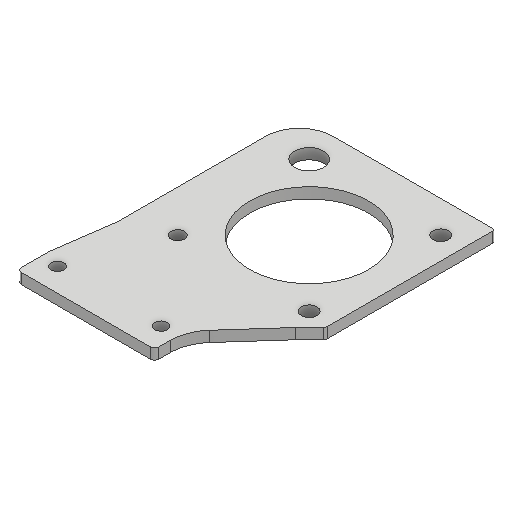
# Autodesk Inventor part: 3DP_ABS_E3D_Titan_Mounting_Plate
Saved by Autodesk Inventor 2026.1 (Build 301233000, 233)
## iProperties
Created: 2017-07-28
Part Number: 3DP_ABS_E3D_Titan_Mounting_Plate
Material: Ogólny
Document SubType Name: Modeling
Designer: Andrzej
Density: 1 g/cm^3
Appearance: Domyślna
Author: Andrzej
Autodesk Inventor part; units mm, degrees
ref_plane "YZ Plane" through (0, 0, 0) normal (1, 0, 0) x (0, 1, 0)
ref_plane "XZ Plane" through (0, 0, 0) normal (0, 1, 0) x (-1, 0, 0)
ref_plane "XY Plane" through (0, 0, 0) normal (0, 0, 1) x (1, 0, 0)
sketch "Szkic1" plane through (0, 0, 0) normal (0, 0, 1) x (1, 0, 0)
  line L0 (-0.9998, 0.9998) -> (-0.9998, 4.2541)
  ellipse E0 centre (0.0003, 1.0002) end of major axis (-0.707, 0.2928) minor radius 1 (-0.9998, 0.9998) -> (0, 0) ccw
  line L1 (0, 0) -> (40.8091, 0)
  ellipse E1 centre (40.809, 1.0002) end of major axis (41.1917, 0.0761) minor radius 1 (40.8091, 0) -> (41.5161, 0.2928) ccw
  line L2 (44.7924, 3.5691) -> (41.5161, 0.2928)
  ellipse E2 centre (44.0851, 4.2762) end of major axis (45.0091, 3.8935) minor radius 1 (44.7924, 3.5691) -> (45.0852, 4.2761) ccw
  line L3 (45.0852, 4.2761) -> (45.0852, 43.2644)
  ellipse E3 centre (44.5851, 43.2643) end of major axis (44.9388, 43.6179) minor radius 0.5 (45.0852, 43.2644) -> (44.5853, 43.7644) ccw
  line L4 (44.5853, 43.7644) -> (6.9989, 43.7644)
  ellipse E4 centre (7.0014, 35.7631) end of major axis (1.3428, 41.4217) minor radius 8 (6.9989, 43.7644) -> (-0.9998, 35.7656) ccw
  line L5 (-0.9998, 7.3746) -> (-0.9998, 35.7656)
  circle A0 centre (24.3209, 20.7644) radius 14
  circle A1 centre (8.8209, 36.2644) radius 3.4
  circle A2 centre (39.8209, 36.2644) radius 1.8356
  circle A3 centre (39.8209, 5.2644) radius 1.8356
  circle A4 centre (8.8209, 5.2644) radius 1.6
  line L6 (-0.9998, 7.3746) -> (-0.9998, 4.2541)
  circle A5 centre (25.4094, -15.2449) radius 1.5
  circle A6 centre (1.0095, -15.2313) radius 1.5
  arc A7 (28.4064, -20.7465) -> (29.4069, -19.7471) centre (28.4069, -19.7465) ccw
  line L7 (29.4106, -13.2471) -> (29.4069, -19.7471)
  line L8 (27.9114, -11.7463) -> (29.4106, -13.2471)
  line L9 (-1.4886, -11.7299) -> (27.9114, -11.7463)
  line L10 (-2.9894, -13.2291) -> (-1.4886, -11.7299)
  line L11 (-2.9931, -19.7291) -> (-2.9894, -13.2291)
  arc A8 (-2.9931, -19.7291) -> (-1.9936, -20.7296) centre (-1.9931, -19.7296) ccw
  line L12 (28.4064, -20.7465) -> (-1.9936, -20.7296)
  line L13 (-2.9894, -13.2291) -> (-0.9998, 0.9998)
  line L14 (29.4106, -13.2471) -> (41.5161, 0.2928)
  point P0 (0, 0)
  point P1 (0, 0)
  dimension "d15" = 0.5001
  dimension "d16" = 1.0002
  dimension "d17" = 1.0002
  dimension "d18" = 8.0024
  dimension "d19" = 1.0003
  dimension "d20" = 0.5
  dimension "d21" = 1
  dimension "d22" = 1
  dimension "d23" = 8
  dimension "d24" = 1
  dimension "d0" = 32.4
  dimension "d1" = 9
  dimension "d2" = 3.5
  dimension "d3" = 3.5
  dimension "d4" = 4
  dimension "d5" = 4
  dimension "d6" = 1
  dimension "d7" = 3
  dimension "d8" = 135
  dimension "d9" = 4.5962
  dimension "d10" = 27.5065
  dimension "d11" = 3.6713
  dimension "d12" = 28
  dimension "d13" = 6.8
  dimension "d14" = 3.2
  dimension "d25" = 135
  dimension "d26" = 46.0851
  dimension "d27" = 43.7644
  dimension "d28" = 45.0852
  dimension "d29" = 29.1492
  dimension "d30" = 43.7644
  dimension "d31" = 4.2761
  dimension "d32" = 3.5691
  dimension "d33" = 5.2644
  dimension "d34" = 26.6344
  dimension "d35" = 5.2644
  dimension "d36" = 4.7141
  dimension "d37" = 20.7644
  dimension "d38" = 26.6344
  dimension "d39" = 20.7644
  dimension "d40" = 26.6344
  dimension "d41" = 36.2644
  dimension "d42" = 48.5547
  dimension "d43" = 36.2644
  dimension "d44" = 26.6344
  dimension "d45" = 45.0852
  dimension "d46" = 29.1492
  dimension "d47" = 35.0709
  dimension "d48" = 32.8644
  dimension "d55" = 11.8
  dimension "d56" = 17
  constraints: 30 end point, 9 centre point, 6 vertical, 4 horizontal, 4 perpendicular, 4 point on circle, 4 tangent, 3 equal radius, 1 collinear, 1 parallel, 23 other
  measures "d0" distance between parallel lines of L11 L7
  measures "d1" distance between parallel lines of L9 L12
  measures "d2" distance from line of L9 A5.centre
  measures "d3" distance from line of L9 A6.centre
  measures "d4" distance from line of L11 A6.centre
  measures "d5" distance from line of L7 A5.centre
  measures "d6" radius of A8
  measures "d7" diameter of A6
  measures "d8" angle of L11 L10
  measures "d9" distance from line of L11.start L10
  measures "d10" distance from line of L11.start L8
  measures "d11" diameter of A2
  measures "d12" diameter of A0
  measures "d13" diameter of A1
  measures "d14" diameter of A4
  measures "d25" angle of L2 L3
  measures "d26" distance between parallel lines of L6 L3
  measures "d27" distance between parallel lines of L1 L4
  measures "d28" distance from line of point (0, 0) L3
  measures "d29" distance from line of point (0, 0) L2
  measures "d30" distance from line of point (0, 0) L4
  measures "d31" distance from line of L3.start L1
  measures "d32" distance from line of L2.end L3
  measures "d33" distance from line of A2.centre L3
  measures "d34" distance from line of A2.centre L2
  measures "d35" distance from line of A3.centre L3
  measures "d36" distance from line of A3.centre L2
  measures "d37" distance from line of A0.centre L3
  measures "d38" distance from line of A0.centre L2
  measures "d39" distance from line of point (24.321, 20.764) L3
  measures "d40" distance from line of point (24.321, 20.764) L2
  measures "d41" distance from line of A1.centre L3
  measures "d42" distance from line of A1.centre L2
  measures "d43" distance from line of A4.centre L3
  measures "d44" distance from line of A4.centre L2
  measures "d45" distance from line of point (0, 0) L3
  measures "d46" distance from line of point (0, 0) L2
  measures "d47" distance from line of L5.start L2
  measures "d48" distance from line of L0.end L2
  measures "d55" distance from line of A4.centre L11
  measures "d56" distance from line of L9 A4.centre
extrude "Wyciągnięcie proste1" add sketch "Szkic1" along normal blind 2.5
fillet "Zaokrąglenie1" radius 10 3 edges at (-2.9931, -19.7291, 1.25) (-0.9998, 0.9998, 1.25) (29.4106, -13.2471, 1.25)
